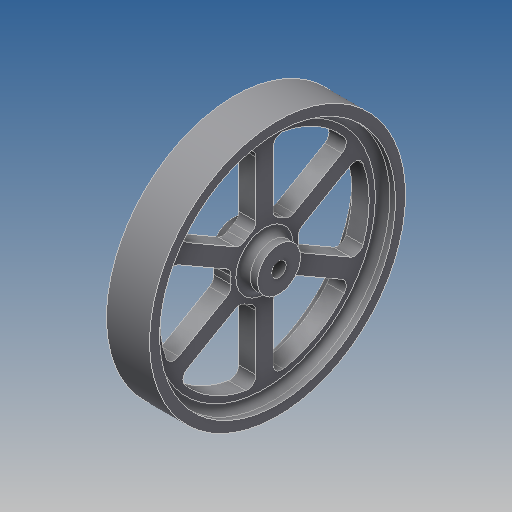
# Autodesk Inventor part: Schwungrad
Saved by Autodesk Inventor 2018 (Build 220112000, 112)
## iProperties
Created: 2018-10-21
Part Number: Schwungrad
Material: Generisch
Document SubType Name: Modeling
Designer: M.Knabel
Density: 1 g/cm^3
Appearance: Vorgabe
Mass: 31.3067 g
Surface Area: 164.53 cm^2
Volume: 31.3067 cm^3
Author: M.Knabel
Autodesk Inventor part; units mm, degrees
ref_plane "XZ Plane" through (0, 0, 0) normal (0, 1, 0) x (-1, 0, 0)
ref_plane "XY Plane" through (0, 0, 0) normal (0, 0, 1) x (1, 0, 0)
sketch "Skizze2" plane through (0, 0, 0) normal (0, 0, 1) x (1, 0, 0)
  line L0 (0, -21.0687) -> (0, 71.4095) projected
  line L1 (-11.2, 0) -> (11.2, 0) projected
  line L2 (-8, 2.5) -> (-8, 7.5)
  line L3 (-5.5, 7.5) -> (-8, 7.5)
  arc A0 (-5.5, 7.5) -> (-3, 10) centre (-5.5, 10) ccw
  line L4 (-3, 10) -> (-3, 38.5)
  arc A1 (-3, 38.5) -> (-5.5, 41) centre (-5.5, 38.5) ccw
  line L5 (-7.5, 44.5) -> (7.5, 44.5)
  line L6 (7.5, 44.5) -> (7.5, 41)
  line L7 (7.5, 41) -> (5.5, 41)
  arc A2 (5.5, 41) -> (3, 38.5) centre (5.5, 38.5) ccw
  line L8 (3, 38.5) -> (3, 10)
  arc A3 (3, 10) -> (5.5, 7.5) centre (5.5, 10) ccw
  line L9 (5.5, 7.5) -> (8, 7.5)
  line L10 (8, 7.5) -> (8, 2.5)
  line L11 (-8, 2.5) -> (8, 2.5)
  line L12 (-7.5, 44.5) -> (-7.5, 41)
  line L13 (-7.5, 41) -> (-5.5, 41)
  line L14 (0, 58.1983) -> (0, -7.8576) construction
  point P0 (0, 0)
  dimension "d5" = 15
  dimension "d7" = 2.5
  dimension "d8" = 2.5
  dimension "d9" = 2.5
  dimension "d10" = 2.5
  dimension "d11" = 89
  dimension "d12" = 82
  dimension "d13" = 15
  dimension "d14" = 6
  dimension "d15" = 7.5
  dimension "d16" = 5
  dimension "d41" = 16
  constraints: 27 end point, 8 point on circle, 8 tangent, 5 perpendicular, 4 centre point, 3 collinear, 3 horizontal, 3 vertical, 2 other
  measures "d5" distance between parallel lines of L6 L12
  measures "d7" radius of A1
  measures "d8" radius of A2
  measures "d9" radius of A3
  measures "d10" radius of A0
  measures "d11" diameter of L5 L1
  measures "d12" diameter of L13 L1
  measures "d13" diameter of L3 L1
  measures "d14" distance between parallel lines of L8 L4
  measures "d15" distance from line of L5.end L14
  measures "d16" diameter of L11 L1
  measures "d41" distance between parallel lines of L10 L2
revolve "Umdrehung1" add sketch "Skizze2" angle 360 about axis through (-10, 0, 0) along (1, 0, 0)
sketch "Skizze3" plane through (-3, 0, 0) normal (-1, 0, 0) x (0, 0, 1)
  line L0 (0, -62.3) -> (0, 62.3) projected
  line L1 (-62.3, 0) -> (62.3, 0) projected
  line L2 (-3.0822, 11.3385) -> (-15.5149, 32.8726)
  line L3 (3.0822, 11.3385) -> (15.5149, 32.8726)
  line L4 (-8.2784, 8.3385) -> (-20.7111, 29.8726)
  line L5 (-36.226, 3) -> (-11.3606, 3)
  line L6 (11.3606, 3) -> (36.226, 3)
  line L7 (8.2784, 8.3385) -> (20.7111, 29.8726)
  line L8 (-3.0822, -11.3385) -> (-15.5149, -32.8726)
  line L9 (3.0822, -11.3385) -> (15.5149, -32.8726)
  line L10 (-8.2784, -8.3385) -> (-20.7111, -29.8726)
  line L11 (-36.226, -3) -> (-11.3606, -3)
  line L12 (11.3606, -3) -> (36.226, -3)
  line L13 (8.2784, -8.3385) -> (20.7111, -29.8726)
  arc A0 (3.0822, 11.3385) -> (-3.0822, 11.3385) centre (0, 0) ccw
  arc A1 (15.5149, 32.8726) -> (-15.5149, 32.8726) centre (0, 0) ccw
  arc A2 (36.226, 3) -> (20.7111, 29.8726) centre (0, 0) ccw
  arc A3 (-20.7111, 29.8726) -> (-36.226, 3) centre (0, 0) ccw
  arc A4 (20.7111, -29.8726) -> (36.226, -3) centre (0, 0) ccw
  arc A5 (-36.226, -3) -> (-20.7111, -29.8726) centre (0, 0) ccw
  arc A6 (-15.5149, -32.8726) -> (15.5149, -32.8726) centre (0, 0) ccw
  arc A7 (-8.2784, 8.3385) -> (-11.3606, 3) centre (0, 0) ccw
  arc A8 (-11.3606, -3) -> (-8.2784, -8.3385) centre (0, 0) ccw
  arc A9 (-3.0822, -11.3385) -> (3.0822, -11.3385) centre (0, 0) ccw
  arc A10 (8.2784, -8.3385) -> (11.3606, -3) centre (0, 0) ccw
  arc A11 (11.3606, 3) -> (8.2784, 8.3385) centre (0, 0) ccw
  dimension "d21" = 60
  dimension "d23" = 6
  dimension "d24" = 6
  dimension "d25" = 3
  dimension "d26" = 3
  dimension "d27" = 60
  dimension "d28" = 36.35
  dimension "d29" = 11.75
  dimension "d30" = 36.35
  dimension "d31" = 11.75
  dimension "d32" = 36.35
  dimension "d33" = 11.75
  constraints: 24 end point, 24 point on circle, 14 symmetric about line, 12 centre point, 4 parallel, 2 coincident, 1 collinear
  measures "d21" angle of L3 L2
  measures "d23" distance between parallel lines of L2 L4
  measures "d24" distance between parallel lines of L7 L3
  measures "d25" distance between parallel lines of L1 L6
  measures "d26" distance between parallel lines of L1 L5
  measures "d27" angle of L5 L4
  measures "d28" radius of A1
  measures "d29" radius of A0
  measures "d30" radius of A2
  measures "d31" radius of A11
  measures "d32" radius of A3
  measures "d33" radius of A7
extrude "Extrusion2" cut sketch "Skizze3" against normal through all
fillet "Rundung1" radius 3 4 edges at (0, 11.3385, -3.0822) (0, 11.3385, 3.0822) (0, 32.8726, -15.5149) (0, 32.8726, 15.5149)
pattern_circular "Runde Anordnung1" count 6 over 360 about axis through (-6.75, 0, 0) along (1, 0, 0) of "Rundung1"
ref_plane "Arbeitsebene1" through (0, 0, 0) normal (0.5, -0.8660254, 0) x (0, 0, 1)
sketch "Skizze5" plane through (0, 0, 0) normal (0.5, -0.8660254, 0) x (0, 0, 1)
  point P0 (0, 0)
  point P1 (0, 0)
  constraints: 1 coincident
hole "Bohrung1" at (0, 0, 0) direction (-0.5, 0.8660254, 0) diameter 2.459 depth 10 tip angle 118 thread size "M3x0.5" class "6H" standard "ISO Metric profile"
